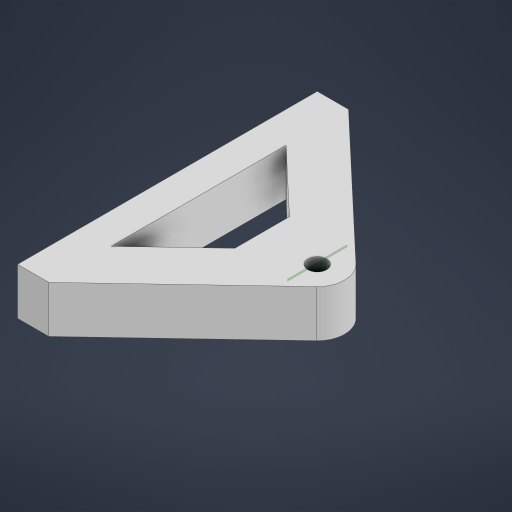
# Autodesk Inventor part: Custom Wheel Mount
Saved by Autodesk Inventor 2023 (Build 270158000, 158)
## iProperties
Created: 2022-10-06
Part Number: Custom Wheel Mount
Material: Generic
Document SubType Name: Modeling
Designer: Izack Waczko
Density: 1 g/cm^3
Appearance: Default
Author: Izack Waczko
Autodesk Inventor part; units mm, degrees
ref_plane "YZ Plane" through (0, 0, 0) normal (1, 0, 0) x (0, 1, 0)
ref_plane "XZ Plane" through (0, 0, 0) normal (0, 1, 0) x (-1, 0, 0)
ref_plane "XY Plane" through (0, 0, 0) normal (0, 0, 1) x (1, 0, 0)
sketch "Sketch1" plane through (0, 0, 0) normal (0, 1, 0) x (-1, 0, 0)
  circle A0 centre (0, 0) radius 3
  circle A1 centre (0, 0) radius 8.75
  line L0 (0, 0) -> (48, 0) construction
  line L1 (48, 48) -> (48, -48) construction
  line L2 (48, 48) -> (38, 48)
  line L3 (38, 48) -> (38, 28)
  line L4 (38, 28) -> (48, 28)
  line L5 (48, 28) -> (48, 48)
  line L6 (38, 48) -> (-6.0137, 6.3559)
  line L7 (38, 28) -> (17.6546, 8.75)
  line L8 (17.6546, 8.75) -> (17.6546, 0)
  line L9 (48, -48) -> (38, -48)
  line L10 (38, -48) -> (38, -28)
  line L11 (38, -28) -> (48, -28)
  line L12 (48, -28) -> (48, -48)
  line L13 (38, -48) -> (-6.0137, -6.3559)
  line L14 (38, -28) -> (17.6546, -8.75)
  line L15 (17.6546, -8.75) -> (17.6546, 0)
  line L16 (48, 28) -> (38, 28)
  line L17 (38, 28) -> (38, -28)
  line L18 (38, -28) -> (48, -28)
  line L19 (48, -28) -> (48, 28)
  dimension "d1" = 17.5
  dimension "d0" = 6
  dimension "d2" = 48
  dimension "d3" = 96
  dimension "d4" = 10
  dimension "d5" = 20
  dimension "d6" = 17.5
  constraints: 40 end point, 5 parallel, 5 symmetric about line, 3 horizontal, 3 perpendicular, 2 coincident, 1 centre point, 1 midpoint, 1 point on line, 1 vertical, 4 other
  measures "d0" diameter of A0
  measures "d2" distance of L0.end L0.start
  measures "d3" distance of L1.start L1.end
  measures "d4" distance of L4.end L3.end
  measures "d5" distance of L2.end L3.end
  measures "d6" distance of L7.end L14.end
extrude "Extrusion1" add sketch "Sketch1" along normal blind 15 contours A1 | A1 L6 L3 L7 L8 L15 L14 L10 L13 | L2 L5 L4 L3 | L10 L11 L12 L9 | L4 L19 L11 L17
ref_plane "Work Plane1" through (0.0004, 0, -8.75) normal (-1, 0, 0) x (0, 0, 1)
body "Solid1"
